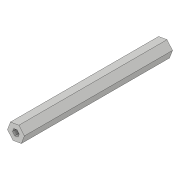
# Autodesk Inventor part: cross beam
Saved by Autodesk Inventor 2018 (Build 220112000, 112)
## iProperties
Created: 2017-12-19
Part Number: cross beam
Material: Generic
Document SubType Name: Modeling
Designer: dsayers
Density: 1 g/cm^3
Appearance: Default
Author: dsayers
Autodesk Inventor part; units mm, degrees
ref_plane "YZ Plane" through (0, 0, 0) normal (1, 0, 0) x (0, 1, 0)
ref_plane "XZ Plane" through (0, 0, 0) normal (0, 1, 0) x (-1, 0, 0)
ref_plane "XY Plane" through (0, 0, 0) normal (0, 0, 1) x (1, 0, 0)
sketch "Sketch1" plane through (0, 0, 0) normal (0, 0, 1) x (1, 0, 0)
  line L0 (2.5344, 6.8804) -> (7.2258, 1.2453)
  line L1 (7.2258, 1.2453) -> (4.6914, -5.6351)
  line L2 (4.6914, -5.6351) -> (-2.5344, -6.8804)
  line L3 (-2.5344, -6.8804) -> (-7.2258, -1.2453)
  line L4 (-7.2258, -1.2453) -> (-4.6914, 5.6351)
  line L5 (-4.6914, 5.6351) -> (2.5344, 6.8804)
  line L6 (-1.847, 2.2185) -> (0.9978, 2.7088)
  line L7 (0.9978, 2.7088) -> (2.8448, 0.4903)
  line L8 (2.8448, 0.4903) -> (1.847, -2.2185)
  line L9 (1.847, -2.2185) -> (-0.9978, -2.7088)
  line L10 (-0.9978, -2.7088) -> (-2.8448, -0.4903)
  line L11 (-2.8448, -0.4903) -> (-1.847, 2.2185)
  point P0 (0, 0)
  point P1 (0, 0)
  point P2 (0, 0)
  dimension "d0" = 12.7
  dimension "d1" = 5
  constraints: 24 end point, 2 coincident, 1 parallel, 26 other
  measures "d0" distance between parallel lines of L2 L5
  measures "d1" distance between parallel lines of L9 L6
extrude "Extrusion1" add sketch "Sketch1" along normal blind 127
body "Solid1"
